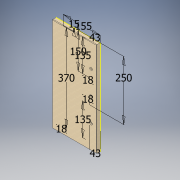
# Autodesk Inventor part: frontHolz
Saved by Autodesk Inventor 2017.2 (Build 212233000, 233)
## iProperties
Part Number: frontHolz
Material: Pappel
Document SubType Name: Modeling
Designer: Daniel
Density: 0.448 g/cm^3
Appearance: Pappel
Author: Daniel
Autodesk Inventor part; units mm, degrees
ref_plane "YZ Plane" through (0, 0, 0) normal (1, 0, 0) x (0, 1, 0)
ref_plane "XZ Plane" through (0, 0, 0) normal (0, 1, 0) x (-1, 0, 0)
ref_plane "XY Plane" through (0, 0, 0) normal (0, 0, 1) x (1, 0, 0)
sketch "Skizze1" plane through (0, 0, 0) normal (0, 1, 0) x (-1, 0, 0)
  line L0 (0, 0) -> (188, 0)
  line L1 (188, 0) -> (188, -400)
  line L2 (188, -400) -> (0, -400)
  line L3 (0, -400) -> (0, 0)
  dimension "d1" = 188
  dimension "d2" = 400
  constraints: 8 end point, 2 parallel, 1 horizontal, 1 perpendicular
  measures "d1" distance of L1.end L2.end
  measures "d2" distance of L0.end L1.end
extrude "Extrusion1" add sketch "Skizze1" along normal blind 15
sketch "Skizze2" plane through (0, 15, 0) normal (0, 1, 0) x (1, 0, 0)
  line L0 (-173, 15) -> (-155, 15)
  line L1 (-155, 15) -> (-155, 385)
  line L2 (-155, 385) -> (-173, 385)
  line L3 (-173, 385) -> (-173, 15)
  line L4 (-43, 15) -> (-61, 15)
  line L5 (-61, 15) -> (-61, 150)
  line L6 (-61, 150) -> (-43, 150)
  line L7 (-43, 150) -> (-43, 15)
  line L8 (-43, 385) -> (-61, 385)
  line L9 (-61, 385) -> (-61, 250)
  line L10 (-61, 250) -> (-43, 250)
  line L11 (-43, 250) -> (-43, 385)
  line L12 (-188, 0) -> (0, 0) projected
  line L13 (0, 0) -> (0, 400) projected
  dimension "d5" = 18
  dimension "d6" = 370
  dimension "d7" = 18
  dimension "d8" = 135
  dimension "d9" = 135
  dimension "d10" = 18
  dimension "d11" = 15
  dimension "d12" = 150
  dimension "d13" = 250
  dimension "d14" = 43
  dimension "d15" = 155
  dimension "d16" = 43
  constraints: 24 end point, 6 parallel, 3 horizontal, 3 perpendicular
  measures "d5" distance of L2.end L1.end
  measures "d6" distance of L1.end L0.end
  measures "d7" distance of L5.end L6.end
  measures "d8" distance of L4.end L5.end
  measures "d9" distance of L9.end L8.end
  measures "d10" distance between parallel lines of L11 L9
  measures "d11" distance between parallel lines of L12 L0
  measures "d12" distance between parallel lines of L12 L6
  measures "d13" distance between parallel lines of L12 L10
  measures "d14" distance between parallel lines of L13 L7
  measures "d15" distance between parallel lines of L13 L1
  measures "d16" distance between parallel lines of L13 L11
extrude "Extrusion2" add sketch "Skizze2" along normal blind 15
sketch "Skizze3" plane through (0, 30, 0) normal (0, 1, 0) x (1, 0, 0)
  point P0 (0, 0)
  point P1 (-52, 45)
  point P2 (-52, 120)
  point P3 (-52, 280)
  point P4 (-52, 355)
  point P5 (-164, 355)
  point P6 (-164, 200)
  point P7 (-164, 45)
hole "Bohrung1" at (-52, 30, -45) at (-52, 30, -120) at (-52, 30, -280) at (-52, 30, -355) at (-164, 30, -355) at (-164, 30, -200) at (-164, 30, -45) direction (0, -1, 0) diameter 4.5 depth 25 tip angle 118 countersink diameter 9 countersink angle 90
sketch "Skizze4" plane through (0, 0, 0) normal (0, -1, 0) x (1, 0, 0)
  line L0 (0, 0) -> (-188, 0) projected
  line L1 (0, -400) -> (0, 0) projected
  point P0 (-23, -200)
  point P1 (-23, -100)
  point P2 (-23, -300)
  dimension "d26" = 100
  dimension "d27" = 200
  dimension "d28" = 300
  dimension "d29" = 23
  dimension "d30" = 23
  dimension "d31" = 23
  measures "d26" distance from line of L0 point (-23, -100)
  measures "d27" distance from line of L0 point (-23, -200)
  measures "d28" distance from line of L0 point (-23, -300)
  measures "d29" distance from line of L1 point (-23, -100)
  measures "d30" distance from line of L1 point (-23, -200)
  measures "d31" distance from line of L1 point (-23, -300)
hole "Bohrung2" at (-23, 0, -100) at (-23, 0, -200) at (-23, 0, -300) direction (0, 1, 0) diameter 6.5 end through all countersink diameter 11.3 countersink angle 90
chamfer "Fase1" distance 2 angle 45 6 edges at (-188, 0, -200) (-94, 0, 0) (-188, 7.5, 0) (0, 0, -200) (-94, 0, -400) (-188, 7.5, -400)
